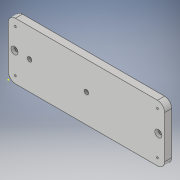
# Autodesk Inventor part: AW5.5aBasePlate
Saved by Autodesk Inventor 2018 (Build 220112000, 112)
## iProperties
Created: 2019-01-17
Part Number: AW5.5aBasePlate
Material: Generic
Document SubType Name: Modeling
Designer: This kid
Density: 1 g/cm^3
Appearance: Default
Author: This kid
Autodesk Inventor part; units mm, degrees
ref_plane "YZ Plane" through (0, 0, 0) normal (1, 0, 0) x (0, 1, 0)
ref_plane "XZ Plane" through (0, 0, 0) normal (0, 1, 0) x (-1, 0, 0)
ref_plane "XY Plane" through (0, 0, 0) normal (0, 0, 1) x (1, 0, 0)
sketch "Sketch1" plane through (0, 0, 0) normal (0, 0, 1) x (1, 0, 0)
  line L0 (12.7, 0) -> (266.7, 0)
  line L1 (279.4, 12.7) -> (279.4, 88.9)
  line L2 (266.7, 101.6) -> (12.7, 101.6)
  line L3 (0, 88.9) -> (0, 12.7)
  arc A0 (3.175, 101.6) -> (0, 98.425) centre (3.175, 98.425) ccw
  arc A1 (266.7, 0) -> (279.4, 12.7) centre (266.7, 12.7) ccw
  arc A2 (12.7, 101.6) -> (0, 88.9) centre (12.7, 88.9) ccw
  arc A3 (0, 12.7) -> (12.7, 0) centre (12.7, 12.7) ccw
  arc A4 (279.4, 88.9) -> (266.7, 101.6) centre (266.7, 88.9) ccw
  point P0 (0, 0)
  point P1 (279.4, 101.6)
  point P2 (279.4, 0)
  point P3 (0, 101.6)
  dimension "d0" = 279.4
  dimension "d1" = 101.6
  dimension "d2" = 3.175
  dimension "d3" = 12.7
  dimension "d28" = 12.7
  constraints: 10 point on circle, 10 point on line, 10 tangent, 8 end point, 5 centre point, 2 equal radius, 2 parallel, 1 horizontal, 1 perpendicular
  measures "d0" distance of point (0, 101.6) point (279.4, 101.6)
  measures "d1" distance of point (279.4, 101.6) point (279.4, 0)
  measures "d2" radius of A0
  measures "d3" radius of A1
  measures "d28" radius of A4
extrude "Extrusion1" add sketch "Sketch1" along normal blind 12.7
sketch "Sketch2" plane through (0, 0, 12.7) normal (0, 0, 1) x (1, 0, 0)
  point P0 (0, 0)
sketch "Sketch3" plane through (0, 0, 12.7) normal (0, 0, 1) x (1, 0, 0)
  line L0 (0, 88.9) -> (0, 12.7) projected
  line L1 (279.4, 12.7) -> (279.4, 88.9) projected
  line L2 (266.7, 101.6) -> (12.7, 101.6) projected
  point P0 (0, 0)
  point P1 (11.0744, 50.8)
  point P2 (38.1, 50.8)
  point P3 (268.2748, 50.8)
  point P4 (139.7, 50.8)
  point P5 (279.4, 101.6)
  dimension "d6" = 11.0744
  dimension "d7" = 38.1
  dimension "d8" = 139.7
  dimension "d9" = 11.1252
  dimension "d10" = 50.8
  dimension "d11" = 50.8
  dimension "d12" = 50.8
  dimension "d13" = 50.8
  measures "d6" distance from line of point (11.074, 50.8) L0
  measures "d7" distance from line of point (38.1, 50.8) L0
  measures "d8" distance from line of point (139.7, 50.8) L0
  measures "d9" distance from line of L1 point (268.275, 50.8)
  measures "d10" distance from line of L2 point (11.074, 50.8)
  measures "d11" distance from line of L2 point (38.1, 50.8)
  measures "d12" distance from line of L2 point (139.7, 50.8)
  measures "d13" distance from line of L2 point (268.275, 50.8)
hole "Hole1" at (11.0744, 50.8, 12.7) at (268.2748, 50.8, 12.7) direction (0, 0, -1) diameter 6.35 end through all countersink diameter 12.7 countersink angle 82
hole "Hole2" at (38.1, 50.8, 12.7) at (139.7, 50.8, 12.7) direction (0, 0, -1) diameter 7.9375 end through all
sketch "Sketch4" plane through (0, 0, 12.7) normal (0, 0, 1) x (1, 0, 0)
  point P0 (0, 0)
sketch "Sketch5" plane through (0, 0, 0) normal (0, 0, -1) x (-1, 0, 0)
  point P0 (0, 0)
hole "Hole3" at (266.7, 88.9, 0) at (266.7, 12.7, 0) at (12.7, 12.7, 0) at (12.7, 88.9, 0) direction (0, 0, 1) diameter 3.302 end through all thread size "8-32 UNC" class "2B" standard "ANSI Unified Screw Threads"
body "Solid1"
